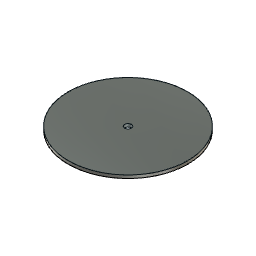
Dial_blank v6 (Autodesk Fusion 360 design; units mm, degrees)
Autodesk Fusion 360 part; units mm, degrees
sketch "Sketch1" plane through (0, 0, 0) normal (0, 0, 1) x (1, 0, 0)
  circle A0 centre (0, 0) radius 14.732
  dimension "d1" = 29.464
  constraint coincident A0.centre origin
  measures "d1" diameter of A0
extrude "Extrude1" add sketch "Sketch1" along normal blind 0.762
sketch "Sketch2" plane through (0, 0, 0.762) normal (0, 0, 1) x (-1, 0, 0)
  circle A0 centre (0, 0) radius 14.732
  circle A1 centre (0, 0) radius 0.8255
  dimension "d4" = 1.651
  constraint coincident A0.centre A1.centre
  measures "d4" diameter of A1
extrude "Extrude2" cut sketch "Sketch2" against normal blind 2.54 contours A1
sketch "Sketch3" plane through (0, 0, 0.762) normal (0, 0, 1) x (-1, 0, 0)
  circle A0 centre (0, 0) radius 0.8255
  circle A1 centre (0, 0) radius 14.732
